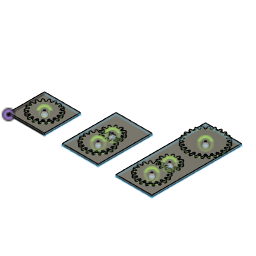
10-dimension-adjust-practice (Autodesk Fusion 360 design; units mm, degrees)
description: Spur Gear; Module: 2.000000; Num Teeth: 18; Pressure Angle: 20.000000; Backlash: 0.00 mm
description: Spur Gear; Module: 2.000000; Num Teeth: 12; Pressure Angle: 20.000000; Backlash: 0.00 mm
description: Spur Gear; Module: 2.000000; Num Teeth: 24; Pressure Angle: 20.000000; Backlash: 0.00 mm
Autodesk Fusion 360 part; units mm, degrees
sketch "スケッチ1" plane through (0, 0, 0) normal (0, 1, 0) x (1, 0, 0)
  line L0 (0, 0) -> (50, 0)
  line L1 (50, 0) -> (50, 50)
  line L2 (50, 50) -> (0, 50)
  line L3 (0, 50) -> (0, 0)
  circle A0 centre (25, 25) radius 1
  line L4 (75, 0) -> (125, 0)
  line L5 (125, 0) -> (125, 75)
  line L6 (125, 75) -> (75, 75)
  line L7 (75, 75) -> (75, 0)
  line L8 (150, 0) -> (200, 0)
  line L9 (200, 0) -> (200, 125)
  line L10 (200, 125) -> (150, 125)
  line L11 (150, 125) -> (150, 0)
  circle A1 centre (100, 25) radius 1
  circle A2 centre (100, 45) radius 1
  circle A3 centre (175, 25) radius 1
  circle A4 centre (175, 50) radius 1
  circle A5 centre (175, 100) radius 1
  dimension "d1" = 2
  dimension "d4" = 2
  dimension "d5" = 2
  dimension "d6" = 2
  dimension "d7" = 2
  dimension "d8" = 2
  constraint horizontal L0
  constraint vertical L1
  constraint horizontal L2
  constraint vertical L3
  constraint coincident L0.start L3.end
  constraint horizontal L4
  constraint vertical L5
  constraint horizontal L6
  constraint vertical L7
  constraint horizontal L8
  constraint vertical L9
  constraint horizontal L10
  constraint vertical L11
  measures "d1" diameter of A0
  measures "d4" diameter of A1
  measures "d5" diameter of A2
  measures "d6" diameter of A3
  measures "d7" diameter of A4
  measures "d8" diameter of A5
extrude "押し出し1" add sketch "スケッチ1" along normal blind 2.5 makes body 1 at (24.9751, 0, -41.9991) makes body 2 at (99.985, 0, -65.333) makes body 3 at (158.0114, 0, -58.4196)
cylinder "円柱プリミティブ2" add diameter 2 height 5 placed x (1, 0, 0) y (0, 0, -1) z (0, 1, 0) at (0, 0, -55) separate body makes body 4
copy_body "ボディ -> コンポーネント1" bodies 1 removing the originals makes body 5 in component "土台1"
copy_body "ボディ -> コンポーネント3" bodies 4 removing the originals makes body 6 in component "軸1"
sketch "スケッチ1 (2)" plane through (0, 0, 0) normal (0, 0, 1) x (1, 0, 0) in component "Spur Gear (18 teeth)"
  circle A0 centre (0, 0) radius 15.5492
  circle A1 centre (0, 0) radius 1
extrude "押し出し1'" add sketch "スケッチ1 (2)" along normal blind 2.5 separate body makes body 7 in component "Spur Gear (18 teeth)"
sketch "スケッチ2" plane through (0, 0, 0) normal (0, 0, 1) x (1, 0, 0) in component "Spur Gear (18 teeth)"
  spline S0 degree 5 poles (16.8263, -1.7252) (16.8353, -1.7261) (16.8534, -1.7277) (16.8805, -1.7293) (16.9168, -1.7301) (16.9623, -1.7292) (17.0078, -1.7268) (17.0533, -1.7236) (17.0989, -1.7199) (17.1446, -1.7159) (17.1902, -1.7115) (17.2359, -1.7067) (17.2816, -1.7013) (17.3273, -1.6953) (17.373, -1.6885) (17.4187, -1.6812) (17.4644, -1.6733) (17.5101, -1.6649) (17.5558, -1.6561) (17.6016, -1.647) (17.6473, -1.6374) (17.693, -1.6275) (17.7387, -1.6172) (17.7844, -1.6064) (17.8301, -1.5952) (17.8757, -1.5836) (17.9214, -1.5716) (17.967, -1.5592) (18.0127, -1.5465) (18.0583, -1.5335) (18.1039, -1.5201) (18.1494, -1.5063) (18.195, -1.4922) (18.2405, -1.4777) (18.286, -1.463) (18.3315, -1.4478) (18.377, -1.4324) (18.4224, -1.4166) (18.4678, -1.4005) (18.5132, -1.3841) (18.5585, -1.3674) (18.6038, -1.3503) (18.6491, -1.333) (18.6943, -1.3153) (18.7396, -1.2974) (18.7847, -1.2791) (18.8299, -1.2606) (18.875, -1.2418) (18.9201, -1.2226) (18.9651, -1.2032) (19.0101, -1.1835) (19.055, -1.1635) (19.1, -1.1433) (19.1448, -1.1227) (19.1897, -1.1019) (19.2344, -1.0808) (19.2792, -1.0594) (19.3239, -1.0378) (19.3685, -1.0159) (19.4131, -0.9937) (19.4577, -0.9712) (19.5022, -0.9485) (19.5467, -0.9255) (19.5911, -0.9023) (19.6354, -0.8788) (19.6797, -0.855) (19.724, -0.831) (19.7682, -0.8067) (19.8123, -0.7822) (19.8564, -0.7574) (19.9005, -0.7324) (19.9357, -0.7122) (19.962, -0.6969) (19.9796, -0.6867) (19.9884, -0.6815) knots 0 0 0 0 0 0 0.01428571 0.02857143 0.04285714 0.05714286 0.07142857 0.08571429 0.1 0.11428571 0.12857143 0.14285714 0.15714286 0.17142857 0.18571429 0.2 0.21428571 0.22857143 0.24285714 0.25714286 0.27142857 0.28571429 0.3 0.31428571 0.32857143 0.34285714 0.35714286 0.37142857 0.38571429 0.4 0.41428571 0.42857143 0.44285714 0.45714286 0.47142857 0.48571429 0.5 0.51428571 0.52857143 0.54285714 0.55714286 0.57142857 0.58571429 0.6 0.61428571 0.62857143 0.64285714 0.65714286 0.67142857 0.68571429 0.7 0.71428571 0.72857143 0.74285714 0.75714286 0.77142857 0.78571429 0.8 0.81428571 0.82857143 0.84285714 0.85714286 0.87142857 0.88571429 0.9 0.91428571 0.92857143 0.94285714 0.95714286 0.97142857 0.98571429 1 1 1 1 1 1
  spline S1 degree 5 poles (16.8263, 1.7252) (16.8353, 1.7261) (16.8534, 1.7277) (16.8805, 1.7293) (16.9168, 1.7301) (16.9623, 1.7292) (17.0078, 1.7268) (17.0533, 1.7236) (17.0989, 1.7199) (17.1446, 1.7159) (17.1902, 1.7115) (17.2359, 1.7067) (17.2816, 1.7013) (17.3273, 1.6953) (17.373, 1.6885) (17.4187, 1.6812) (17.4644, 1.6733) (17.5101, 1.6649) (17.5558, 1.6561) (17.6016, 1.647) (17.6473, 1.6374) (17.693, 1.6275) (17.7387, 1.6172) (17.7844, 1.6064) (17.8301, 1.5952) (17.8757, 1.5836) (17.9214, 1.5716) (17.967, 1.5592) (18.0127, 1.5465) (18.0583, 1.5335) (18.1039, 1.5201) (18.1494, 1.5063) (18.195, 1.4922) (18.2405, 1.4777) (18.286, 1.463) (18.3315, 1.4478) (18.377, 1.4324) (18.4224, 1.4166) (18.4678, 1.4005) (18.5132, 1.3841) (18.5585, 1.3674) (18.6038, 1.3503) (18.6491, 1.333) (18.6943, 1.3153) (18.7396, 1.2974) (18.7847, 1.2791) (18.8299, 1.2606) (18.875, 1.2418) (18.9201, 1.2226) (18.9651, 1.2032) (19.0101, 1.1835) (19.055, 1.1635) (19.1, 1.1433) (19.1448, 1.1227) (19.1897, 1.1019) (19.2344, 1.0808) (19.2792, 1.0594) (19.3239, 1.0378) (19.3685, 1.0159) (19.4131, 0.9937) (19.4577, 0.9712) (19.5022, 0.9485) (19.5467, 0.9255) (19.5911, 0.9023) (19.6354, 0.8788) (19.6797, 0.855) (19.724, 0.831) (19.7682, 0.8067) (19.8123, 0.7822) (19.8564, 0.7574) (19.9005, 0.7324) (19.9357, 0.7122) (19.962, 0.6969) (19.9796, 0.6867) (19.9884, 0.6815) knots 0 0 0 0 0 0 0.01428571 0.02857143 0.04285714 0.05714286 0.07142857 0.08571429 0.1 0.11428571 0.12857143 0.14285714 0.15714286 0.17142857 0.18571429 0.2 0.21428571 0.22857143 0.24285714 0.25714286 0.27142857 0.28571429 0.3 0.31428571 0.32857143 0.34285714 0.35714286 0.37142857 0.38571429 0.4 0.41428571 0.42857143 0.44285714 0.45714286 0.47142857 0.48571429 0.5 0.51428571 0.52857143 0.54285714 0.55714286 0.57142857 0.58571429 0.6 0.61428571 0.62857143 0.64285714 0.65714286 0.67142857 0.68571429 0.7 0.71428571 0.72857143 0.74285714 0.75714286 0.77142857 0.78571429 0.8 0.81428571 0.82857143 0.84285714 0.85714286 0.87142857 0.88571429 0.9 0.91428571 0.92857143 0.94285714 0.95714286 0.97142857 0.98571429 1 1 1 1 1 1
  arc A0 (19.9884, -0.6815) -> (19.9884, 0.6815) centre (0, 0) ccw
  line L0 (15.4582, -1.5859) -> (16.8263, -1.7252)
  line L1 (15.4582, 1.5859) -> (16.8263, 1.7252)
  line L2 (15.4582, -1.5859) -> (15.4582, 1.5859)
  point P0 (17.0479, -1.7239)
  point P1 (17.2716, -1.7024)
  point P2 (17.4964, -1.6673)
  point P3 (17.7221, -1.6209)
  point P4 (17.9484, -1.5642)
  point P5 (18.1752, -1.4983)
  point P6 (18.4023, -1.4236)
  point P7 (18.6295, -1.3405)
  point P8 (18.8567, -1.2494)
  point P9 (19.0838, -1.1505)
  point P10 (19.3106, -1.0442)
  point P11 (19.5371, -0.9304)
  point P12 (19.763, -0.8095)
  point P13 (17.0479, 1.7239)
  point P14 (17.2716, 1.7024)
  point P15 (17.4964, 1.6673)
  point P16 (17.7221, 1.6209)
  point P17 (17.9484, 1.5642)
  point P18 (18.1752, 1.4983)
  point P19 (18.4023, 1.4236)
  point P20 (18.6295, 1.3405)
  point P21 (18.8567, 1.2494)
  point P22 (19.0838, 1.1505)
  point P23 (19.3106, 1.0442)
  point P24 (19.5371, 0.9304)
  point P25 (19.763, 0.8095)
extrude "押し出し2" add sketch "スケッチ2" along normal blind 2.5 bodies 7 in component "Spur Gear (18 teeth)"
fillet "フィレット1" radius 1 2 edges at (15.468, -1.5869, 1.25) (15.468, 1.5869, 1.25) on bodies 7 in component "Spur Gear (18 teeth)"
pattern_circular "C パターン1" count 18 over 360 about axis through (0, 0, 0) along (0, 0, 1) of "押し出し2", "フィレット1" in component "Spur Gear (18 teeth)"
sketch "スケッチ3" plane through (0, 0, 0) normal (0, 0, 1) x (1, 0, 0) in component "Spur Gear (18 teeth)"
  circle A0 centre (0, 0) radius 18 construction
cylinder "円柱プリミティブ3" add diameter 2 height 5 placed x (1, 0, 0) y (0, 0, -1) z (0, 1, 0) at (75, 0, -80) separate body makes body 8
copy_body "ボディ -> コンポーネント4" bodies 2 removing the originals makes body 9 in component "土台2"
copy_body "ボディ -> コンポーネント5" bodies 8 removing the originals makes body 10 in component "軸2"
sketch "スケッチ1 (3)" plane through (0, 0, 0) normal (0, 0, 1) x (1, 0, 0) in component "Spur Gear (18 teeth) (1)"
  circle A0 centre (0, 0) radius 15.5492
  circle A1 centre (0, 0) radius 1
extrude "押し出し1''" add sketch "スケッチ1 (3)" along normal blind 2.5 separate body makes body 11 in component "Spur Gear (18 teeth) (1)"
sketch "スケッチ2 (2)" plane through (0, 0, 0) normal (0, 0, 1) x (1, 0, 0) in component "Spur Gear (18 teeth) (1)"
  spline S0 degree 5 poles (16.8263, -1.7252) (16.8353, -1.7261) (16.8534, -1.7277) (16.8805, -1.7293) (16.9168, -1.7301) (16.9623, -1.7292) (17.0078, -1.7268) (17.0533, -1.7236) (17.0989, -1.7199) (17.1446, -1.7159) (17.1902, -1.7115) (17.2359, -1.7067) (17.2816, -1.7013) (17.3273, -1.6953) (17.373, -1.6885) (17.4187, -1.6812) (17.4644, -1.6733) (17.5101, -1.6649) (17.5558, -1.6561) (17.6016, -1.647) (17.6473, -1.6374) (17.693, -1.6275) (17.7387, -1.6172) (17.7844, -1.6064) (17.8301, -1.5952) (17.8757, -1.5836) (17.9214, -1.5716) (17.967, -1.5592) (18.0127, -1.5465) (18.0583, -1.5335) (18.1039, -1.5201) (18.1494, -1.5063) (18.195, -1.4922) (18.2405, -1.4777) (18.286, -1.463) (18.3315, -1.4478) (18.377, -1.4324) (18.4224, -1.4166) (18.4678, -1.4005) (18.5132, -1.3841) (18.5585, -1.3674) (18.6038, -1.3503) (18.6491, -1.333) (18.6943, -1.3153) (18.7396, -1.2974) (18.7847, -1.2791) (18.8299, -1.2606) (18.875, -1.2418) (18.9201, -1.2226) (18.9651, -1.2032) (19.0101, -1.1835) (19.055, -1.1635) (19.1, -1.1433) (19.1448, -1.1227) (19.1897, -1.1019) (19.2344, -1.0808) (19.2792, -1.0594) (19.3239, -1.0378) (19.3685, -1.0159) (19.4131, -0.9937) (19.4577, -0.9712) (19.5022, -0.9485) (19.5467, -0.9255) (19.5911, -0.9023) (19.6354, -0.8788) (19.6797, -0.855) (19.724, -0.831) (19.7682, -0.8067) (19.8123, -0.7822) (19.8564, -0.7574) (19.9005, -0.7324) (19.9357, -0.7122) (19.962, -0.6969) (19.9796, -0.6867) (19.9884, -0.6815) knots 0 0 0 0 0 0 0.01428571 0.02857143 0.04285714 0.05714286 0.07142857 0.08571429 0.1 0.11428571 0.12857143 0.14285714 0.15714286 0.17142857 0.18571429 0.2 0.21428571 0.22857143 0.24285714 0.25714286 0.27142857 0.28571429 0.3 0.31428571 0.32857143 0.34285714 0.35714286 0.37142857 0.38571429 0.4 0.41428571 0.42857143 0.44285714 0.45714286 0.47142857 0.48571429 0.5 0.51428571 0.52857143 0.54285714 0.55714286 0.57142857 0.58571429 0.6 0.61428571 0.62857143 0.64285714 0.65714286 0.67142857 0.68571429 0.7 0.71428571 0.72857143 0.74285714 0.75714286 0.77142857 0.78571429 0.8 0.81428571 0.82857143 0.84285714 0.85714286 0.87142857 0.88571429 0.9 0.91428571 0.92857143 0.94285714 0.95714286 0.97142857 0.98571429 1 1 1 1 1 1
  spline S1 degree 5 poles (16.8263, 1.7252) (16.8353, 1.7261) (16.8534, 1.7277) (16.8805, 1.7293) (16.9168, 1.7301) (16.9623, 1.7292) (17.0078, 1.7268) (17.0533, 1.7236) (17.0989, 1.7199) (17.1446, 1.7159) (17.1902, 1.7115) (17.2359, 1.7067) (17.2816, 1.7013) (17.3273, 1.6953) (17.373, 1.6885) (17.4187, 1.6812) (17.4644, 1.6733) (17.5101, 1.6649) (17.5558, 1.6561) (17.6016, 1.647) (17.6473, 1.6374) (17.693, 1.6275) (17.7387, 1.6172) (17.7844, 1.6064) (17.8301, 1.5952) (17.8757, 1.5836) (17.9214, 1.5716) (17.967, 1.5592) (18.0127, 1.5465) (18.0583, 1.5335) (18.1039, 1.5201) (18.1494, 1.5063) (18.195, 1.4922) (18.2405, 1.4777) (18.286, 1.463) (18.3315, 1.4478) (18.377, 1.4324) (18.4224, 1.4166) (18.4678, 1.4005) (18.5132, 1.3841) (18.5585, 1.3674) (18.6038, 1.3503) (18.6491, 1.333) (18.6943, 1.3153) (18.7396, 1.2974) (18.7847, 1.2791) (18.8299, 1.2606) (18.875, 1.2418) (18.9201, 1.2226) (18.9651, 1.2032) (19.0101, 1.1835) (19.055, 1.1635) (19.1, 1.1433) (19.1448, 1.1227) (19.1897, 1.1019) (19.2344, 1.0808) (19.2792, 1.0594) (19.3239, 1.0378) (19.3685, 1.0159) (19.4131, 0.9937) (19.4577, 0.9712) (19.5022, 0.9485) (19.5467, 0.9255) (19.5911, 0.9023) (19.6354, 0.8788) (19.6797, 0.855) (19.724, 0.831) (19.7682, 0.8067) (19.8123, 0.7822) (19.8564, 0.7574) (19.9005, 0.7324) (19.9357, 0.7122) (19.962, 0.6969) (19.9796, 0.6867) (19.9884, 0.6815) knots 0 0 0 0 0 0 0.01428571 0.02857143 0.04285714 0.05714286 0.07142857 0.08571429 0.1 0.11428571 0.12857143 0.14285714 0.15714286 0.17142857 0.18571429 0.2 0.21428571 0.22857143 0.24285714 0.25714286 0.27142857 0.28571429 0.3 0.31428571 0.32857143 0.34285714 0.35714286 0.37142857 0.38571429 0.4 0.41428571 0.42857143 0.44285714 0.45714286 0.47142857 0.48571429 0.5 0.51428571 0.52857143 0.54285714 0.55714286 0.57142857 0.58571429 0.6 0.61428571 0.62857143 0.64285714 0.65714286 0.67142857 0.68571429 0.7 0.71428571 0.72857143 0.74285714 0.75714286 0.77142857 0.78571429 0.8 0.81428571 0.82857143 0.84285714 0.85714286 0.87142857 0.88571429 0.9 0.91428571 0.92857143 0.94285714 0.95714286 0.97142857 0.98571429 1 1 1 1 1 1
  arc A0 (19.9884, -0.6815) -> (19.9884, 0.6815) centre (0, 0) ccw
  line L0 (15.4582, -1.5859) -> (16.8263, -1.7252)
  line L1 (15.4582, 1.5859) -> (16.8263, 1.7252)
  line L2 (15.4582, -1.5859) -> (15.4582, 1.5859)
  point P0 (17.0479, -1.7239)
  point P1 (17.2716, -1.7024)
  point P2 (17.4964, -1.6673)
  point P3 (17.7221, -1.6209)
  point P4 (17.9484, -1.5642)
  point P5 (18.1752, -1.4983)
  point P6 (18.4023, -1.4236)
  point P7 (18.6295, -1.3405)
  point P8 (18.8567, -1.2494)
  point P9 (19.0838, -1.1505)
  point P10 (19.3106, -1.0442)
  point P11 (19.5371, -0.9304)
  point P12 (19.763, -0.8095)
  point P13 (17.0479, 1.7239)
  point P14 (17.2716, 1.7024)
  point P15 (17.4964, 1.6673)
  point P16 (17.7221, 1.6209)
  point P17 (17.9484, 1.5642)
  point P18 (18.1752, 1.4983)
  point P19 (18.4023, 1.4236)
  point P20 (18.6295, 1.3405)
  point P21 (18.8567, 1.2494)
  point P22 (19.0838, 1.1505)
  point P23 (19.3106, 1.0442)
  point P24 (19.5371, 0.9304)
  point P25 (19.763, 0.8095)
extrude "押し出し2'" add sketch "スケッチ2 (2)" along normal blind 2.5 bodies 11 in component "Spur Gear (18 teeth) (1)"
fillet "フィレット1'" radius 1 2 edges at (15.468, -1.5869, 1.25) (15.468, 1.5869, 1.25) on bodies 11 in component "Spur Gear (18 teeth) (1)"
pattern_circular "C パターン1'" count 18 over 360 about axis through (0, 0, 0) along (0, 0, 1) of "押し出し2'", "フィレット1'" in component "Spur Gear (18 teeth) (1)"
sketch "スケッチ3 (2)" plane through (0, 0, 0) normal (0, 0, 1) x (1, 0, 0) in component "Spur Gear (18 teeth) (1)"
  circle A0 centre (0, 0) radius 18 construction
sketch "スケッチ1 (4)" plane through (0, 0, 0) normal (0, 0, 1) x (1, 0, 0) in component "Spur Gear (12 teeth)"
  circle A0 centre (0, 0) radius 9.5492
  circle A1 centre (0, 0) radius 1
extrude "押し出し1'''" add sketch "スケッチ1 (4)" along normal blind 2.5 separate body makes body 12 in component "Spur Gear (12 teeth)"
sketch "スケッチ2 (3)" plane through (0, 0, 0) normal (0, 0, 1) x (1, 0, 0) in component "Spur Gear (12 teeth)"
  spline S0 degree 5 poles (11.1567, -1.6383) (11.1647, -1.6395) (11.1807, -1.6416) (11.2048, -1.6439) (11.237, -1.6456) (11.2774, -1.6458) (11.318, -1.6445) (11.3587, -1.6423) (11.3994, -1.6396) (11.4401, -1.6366) (11.4809, -1.6333) (11.5218, -1.6295) (11.5626, -1.625) (11.6035, -1.6199) (11.6445, -1.614) (11.6854, -1.6075) (11.7264, -1.6005) (11.7674, -1.5929) (11.8084, -1.585) (11.8494, -1.5766) (11.8905, -1.5678) (11.9315, -1.5587) (11.9725, -1.5491) (12.0135, -1.539) (12.0545, -1.5285) (12.0956, -1.5175) (12.1366, -1.5062) (12.1776, -1.4944) (12.2186, -1.4823) (12.2595, -1.4698) (12.3005, -1.4569) (12.3414, -1.4437) (12.3824, -1.4301) (12.4233, -1.4161) (12.4641, -1.4018) (12.505, -1.3871) (12.5458, -1.372) (12.5866, -1.3566) (12.6274, -1.3409) (12.6681, -1.3248) (12.7088, -1.3084) (12.7495, -1.2917) (12.7902, -1.2746) (12.8308, -1.2572) (12.8713, -1.2395) (12.9119, -1.2215) (12.9523, -1.2031) (12.9928, -1.1844) (13.0332, -1.1654) (13.0735, -1.1461) (13.1138, -1.1265) (13.1541, -1.1066) (13.1943, -1.0863) (13.2345, -1.0658) (13.2746, -1.045) (13.3146, -1.0239) (13.3546, -1.0024) (13.3946, -0.9807) (13.4344, -0.9587) (13.4743, -0.9364) (13.514, -0.9138) (13.5538, -0.8909) (13.5934, -0.8678) (13.633, -0.8443) (13.6725, -0.8206) (13.712, -0.7966) (13.7514, -0.7723) (13.7907, -0.7477) (13.8299, -0.7229) (13.8691, -0.6978) (13.9082, -0.6724) (13.9395, -0.6518) (13.9629, -0.6363) (13.9784, -0.6259) (13.9862, -0.6207) knots 0 0 0 0 0 0 0.01428571 0.02857143 0.04285714 0.05714286 0.07142857 0.08571429 0.1 0.11428571 0.12857143 0.14285714 0.15714286 0.17142857 0.18571429 0.2 0.21428571 0.22857143 0.24285714 0.25714286 0.27142857 0.28571429 0.3 0.31428571 0.32857143 0.34285714 0.35714286 0.37142857 0.38571429 0.4 0.41428571 0.42857143 0.44285714 0.45714286 0.47142857 0.48571429 0.5 0.51428571 0.52857143 0.54285714 0.55714286 0.57142857 0.58571429 0.6 0.61428571 0.62857143 0.64285714 0.65714286 0.67142857 0.68571429 0.7 0.71428571 0.72857143 0.74285714 0.75714286 0.77142857 0.78571429 0.8 0.81428571 0.82857143 0.84285714 0.85714286 0.87142857 0.88571429 0.9 0.91428571 0.92857143 0.94285714 0.95714286 0.97142857 0.98571429 1 1 1 1 1 1
  spline S1 degree 5 poles (11.1567, 1.6383) (11.1647, 1.6395) (11.1807, 1.6416) (11.2048, 1.6439) (11.237, 1.6456) (11.2774, 1.6458) (11.318, 1.6445) (11.3587, 1.6423) (11.3994, 1.6396) (11.4401, 1.6366) (11.4809, 1.6333) (11.5218, 1.6295) (11.5626, 1.625) (11.6035, 1.6199) (11.6445, 1.614) (11.6854, 1.6075) (11.7264, 1.6005) (11.7674, 1.5929) (11.8084, 1.585) (11.8494, 1.5766) (11.8905, 1.5678) (11.9315, 1.5587) (11.9725, 1.5491) (12.0135, 1.539) (12.0545, 1.5285) (12.0956, 1.5175) (12.1366, 1.5062) (12.1776, 1.4944) (12.2186, 1.4823) (12.2595, 1.4698) (12.3005, 1.4569) (12.3414, 1.4437) (12.3824, 1.4301) (12.4233, 1.4161) (12.4641, 1.4018) (12.505, 1.3871) (12.5458, 1.372) (12.5866, 1.3566) (12.6274, 1.3409) (12.6681, 1.3248) (12.7088, 1.3084) (12.7495, 1.2917) (12.7902, 1.2746) (12.8308, 1.2572) (12.8713, 1.2395) (12.9119, 1.2215) (12.9523, 1.2031) (12.9928, 1.1844) (13.0332, 1.1654) (13.0735, 1.1461) (13.1138, 1.1265) (13.1541, 1.1066) (13.1943, 1.0863) (13.2345, 1.0658) (13.2746, 1.045) (13.3146, 1.0239) (13.3546, 1.0024) (13.3946, 0.9807) (13.4344, 0.9587) (13.4743, 0.9364) (13.514, 0.9138) (13.5538, 0.8909) (13.5934, 0.8678) (13.633, 0.8443) (13.6725, 0.8206) (13.712, 0.7966) (13.7514, 0.7723) (13.7907, 0.7477) (13.8299, 0.7229) (13.8691, 0.6978) (13.9082, 0.6724) (13.9395, 0.6518) (13.9629, 0.6363) (13.9784, 0.6259) (13.9862, 0.6207) knots 0 0 0 0 0 0 0.01428571 0.02857143 0.04285714 0.05714286 0.07142857 0.08571429 0.1 0.11428571 0.12857143 0.14285714 0.15714286 0.17142857 0.18571429 0.2 0.21428571 0.22857143 0.24285714 0.25714286 0.27142857 0.28571429 0.3 0.31428571 0.32857143 0.34285714 0.35714286 0.37142857 0.38571429 0.4 0.41428571 0.42857143 0.44285714 0.45714286 0.47142857 0.48571429 0.5 0.51428571 0.52857143 0.54285714 0.55714286 0.57142857 0.58571429 0.6 0.61428571 0.62857143 0.64285714 0.65714286 0.67142857 0.68571429 0.7 0.71428571 0.72857143 0.74285714 0.75714286 0.77142857 0.78571429 0.8 0.81428571 0.82857143 0.84285714 0.85714286 0.87142857 0.88571429 0.9 0.91428571 0.92857143 0.94285714 0.95714286 0.97142857 0.98571429 1 1 1 1 1 1
  arc A0 (13.9862, -0.6207) -> (13.9862, 0.6207) centre (0, 0) ccw
  line L0 (9.438, -1.3874) -> (11.1567, -1.6383)
  line L1 (9.438, 1.3874) -> (11.1567, 1.6383)
  line L2 (9.438, -1.3874) -> (9.438, 1.3874)
  point P0 (11.3527, -1.6425)
  point P1 (11.5515, -1.6261)
  point P2 (11.7521, -1.5957)
  point P3 (11.954, -1.5533)
  point P4 (12.1568, -1.5003)
  point P5 (12.3603, -1.4374)
  point P6 (12.5642, -1.3651)
  point P7 (12.7683, -1.2838)
  point P8 (12.9724, -1.1938)
  point P9 (13.1764, -1.0953)
  point P10 (13.3799, -0.9887)
  point P11 (13.5828, -0.8739)
  point P12 (13.785, -0.7512)
  point P13 (11.3527, 1.6425)
  point P14 (11.5515, 1.6261)
  point P15 (11.7521, 1.5957)
  point P16 (11.954, 1.5533)
  point P17 (12.1568, 1.5003)
  point P18 (12.3603, 1.4374)
  point P19 (12.5642, 1.3651)
  point P20 (12.7683, 1.2838)
  point P21 (12.9724, 1.1938)
  point P22 (13.1764, 1.0953)
  point P23 (13.3799, 0.9887)
  point P24 (13.5828, 0.8739)
  point P25 (13.785, 0.7512)
extrude "押し出し2''" add sketch "スケッチ2 (3)" along normal blind 2.5 bodies 12 in component "Spur Gear (12 teeth)"
fillet "フィレット1''" radius 1 2 edges at (9.4477, -1.3888, 1.25) (9.4477, 1.3888, 1.25) on bodies 12 in component "Spur Gear (12 teeth)"
pattern_circular "C パターン1''" count 12 over 360 about axis through (0, 0, 0) along (0, 0, 1) of "押し出し2''", "フィレット1''" in component "Spur Gear (12 teeth)"
sketch "スケッチ3 (3)" plane through (0, 0, 0) normal (0, 0, 1) x (1, 0, 0) in component "Spur Gear (12 teeth)"
  circle A0 centre (0, 0) radius 12 construction
cylinder "円柱プリミティブ4" add diameter 2 height 5 placed x (1, 0, 0) y (0, 0, -1) z (0, 1, 0) at (150, 0, -130) separate body makes body 13
copy_body "ボディ -> コンポーネント7" bodies 13 removing the originals makes body 14 in component "軸3"
copy_body "ボディ -> コンポーネント8" bodies 3 removing the originals makes body 15 in component "土台3"
sketch "スケッチ1 (5)" plane through (0, 0, 0) normal (0, 0, 1) x (1, 0, 0) in component "Spur Gear (18 teeth) (2)"
  circle A0 centre (0, 0) radius 15.5492
  circle A1 centre (0, 0) radius 1
extrude "押し出し1''''" add sketch "スケッチ1 (5)" along normal blind 2.5 separate body makes body 16 in component "Spur Gear (18 teeth) (2)"
sketch "スケッチ2 (4)" plane through (0, 0, 0) normal (0, 0, 1) x (1, 0, 0) in component "Spur Gear (18 teeth) (2)"
  spline S0 degree 5 poles (16.8263, -1.7252) (16.8353, -1.7261) (16.8534, -1.7277) (16.8805, -1.7293) (16.9168, -1.7301) (16.9623, -1.7292) (17.0078, -1.7268) (17.0533, -1.7236) (17.0989, -1.7199) (17.1446, -1.7159) (17.1902, -1.7115) (17.2359, -1.7067) (17.2816, -1.7013) (17.3273, -1.6953) (17.373, -1.6885) (17.4187, -1.6812) (17.4644, -1.6733) (17.5101, -1.6649) (17.5558, -1.6561) (17.6016, -1.647) (17.6473, -1.6374) (17.693, -1.6275) (17.7387, -1.6172) (17.7844, -1.6064) (17.8301, -1.5952) (17.8757, -1.5836) (17.9214, -1.5716) (17.967, -1.5592) (18.0127, -1.5465) (18.0583, -1.5335) (18.1039, -1.5201) (18.1494, -1.5063) (18.195, -1.4922) (18.2405, -1.4777) (18.286, -1.463) (18.3315, -1.4478) (18.377, -1.4324) (18.4224, -1.4166) (18.4678, -1.4005) (18.5132, -1.3841) (18.5585, -1.3674) (18.6038, -1.3503) (18.6491, -1.333) (18.6943, -1.3153) (18.7396, -1.2974) (18.7847, -1.2791) (18.8299, -1.2606) (18.875, -1.2418) (18.9201, -1.2226) (18.9651, -1.2032) (19.0101, -1.1835) (19.055, -1.1635) (19.1, -1.1433) (19.1448, -1.1227) (19.1897, -1.1019) (19.2344, -1.0808) (19.2792, -1.0594) (19.3239, -1.0378) (19.3685, -1.0159) (19.4131, -0.9937) (19.4577, -0.9712) (19.5022, -0.9485) (19.5467, -0.9255) (19.5911, -0.9023) (19.6354, -0.8788) (19.6797, -0.855) (19.724, -0.831) (19.7682, -0.8067) (19.8123, -0.7822) (19.8564, -0.7574) (19.9005, -0.7324) (19.9357, -0.7122) (19.962, -0.6969) (19.9796, -0.6867) (19.9884, -0.6815) knots 0 0 0 0 0 0 0.01428571 0.02857143 0.04285714 0.05714286 0.07142857 0.08571429 0.1 0.11428571 0.12857143 0.14285714 0.15714286 0.17142857 0.18571429 0.2 0.21428571 0.22857143 0.24285714 0.25714286 0.27142857 0.28571429 0.3 0.31428571 0.32857143 0.34285714 0.35714286 0.37142857 0.38571429 0.4 0.41428571 0.42857143 0.44285714 0.45714286 0.47142857 0.48571429 0.5 0.51428571 0.52857143 0.54285714 0.55714286 0.57142857 0.58571429 0.6 0.61428571 0.62857143 0.64285714 0.65714286 0.67142857 0.68571429 0.7 0.71428571 0.72857143 0.74285714 0.75714286 0.77142857 0.78571429 0.8 0.81428571 0.82857143 0.84285714 0.85714286 0.87142857 0.88571429 0.9 0.91428571 0.92857143 0.94285714 0.95714286 0.97142857 0.98571429 1 1 1 1 1 1
  spline S1 degree 5 poles (16.8263, 1.7252) (16.8353, 1.7261) (16.8534, 1.7277) (16.8805, 1.7293) (16.9168, 1.7301) (16.9623, 1.7292) (17.0078, 1.7268) (17.0533, 1.7236) (17.0989, 1.7199) (17.1446, 1.7159) (17.1902, 1.7115) (17.2359, 1.7067) (17.2816, 1.7013) (17.3273, 1.6953) (17.373, 1.6885) (17.4187, 1.6812) (17.4644, 1.6733) (17.5101, 1.6649) (17.5558, 1.6561) (17.6016, 1.647) (17.6473, 1.6374) (17.693, 1.6275) (17.7387, 1.6172) (17.7844, 1.6064) (17.8301, 1.5952) (17.8757, 1.5836) (17.9214, 1.5716) (17.967, 1.5592) (18.0127, 1.5465) (18.0583, 1.5335) (18.1039, 1.5201) (18.1494, 1.5063) (18.195, 1.4922) (18.2405, 1.4777) (18.286, 1.463) (18.3315, 1.4478) (18.377, 1.4324) (18.4224, 1.4166) (18.4678, 1.4005) (18.5132, 1.3841) (18.5585, 1.3674) (18.6038, 1.3503) (18.6491, 1.333) (18.6943, 1.3153) (18.7396, 1.2974) (18.7847, 1.2791) (18.8299, 1.2606) (18.875, 1.2418) (18.9201, 1.2226) (18.9651, 1.2032) (19.0101, 1.1835) (19.055, 1.1635) (19.1, 1.1433) (19.1448, 1.1227) (19.1897, 1.1019) (19.2344, 1.0808) (19.2792, 1.0594) (19.3239, 1.0378) (19.3685, 1.0159) (19.4131, 0.9937) (19.4577, 0.9712) (19.5022, 0.9485) (19.5467, 0.9255) (19.5911, 0.9023) (19.6354, 0.8788) (19.6797, 0.855) (19.724, 0.831) (19.7682, 0.8067) (19.8123, 0.7822) (19.8564, 0.7574) (19.9005, 0.7324) (19.9357, 0.7122) (19.962, 0.6969) (19.9796, 0.6867) (19.9884, 0.6815) knots 0 0 0 0 0 0 0.01428571 0.02857143 0.04285714 0.05714286 0.07142857 0.08571429 0.1 0.11428571 0.12857143 0.14285714 0.15714286 0.17142857 0.18571429 0.2 0.21428571 0.22857143 0.24285714 0.25714286 0.27142857 0.28571429 0.3 0.31428571 0.32857143 0.34285714 0.35714286 0.37142857 0.38571429 0.4 0.41428571 0.42857143 0.44285714 0.45714286 0.47142857 0.48571429 0.5 0.51428571 0.52857143 0.54285714 0.55714286 0.57142857 0.58571429 0.6 0.61428571 0.62857143 0.64285714 0.65714286 0.67142857 0.68571429 0.7 0.71428571 0.72857143 0.74285714 0.75714286 0.77142857 0.78571429 0.8 0.81428571 0.82857143 0.84285714 0.85714286 0.87142857 0.88571429 0.9 0.91428571 0.92857143 0.94285714 0.95714286 0.97142857 0.98571429 1 1 1 1 1 1
  arc A0 (19.9884, -0.6815) -> (19.9884, 0.6815) centre (0, 0) ccw
  line L0 (15.4582, -1.5859) -> (16.8263, -1.7252)
  line L1 (15.4582, 1.5859) -> (16.8263, 1.7252)
  line L2 (15.4582, -1.5859) -> (15.4582, 1.5859)
  point P0 (17.0479, -1.7239)
  point P1 (17.2716, -1.7024)
  point P2 (17.4964, -1.6673)
  point P3 (17.7221, -1.6209)
  point P4 (17.9484, -1.5642)
  point P5 (18.1752, -1.4983)
  point P6 (18.4023, -1.4236)
  point P7 (18.6295, -1.3405)
  point P8 (18.8567, -1.2494)
  point P9 (19.0838, -1.1505)
  point P10 (19.3106, -1.0442)
  point P11 (19.5371, -0.9304)
  point P12 (19.763, -0.8095)
  point P13 (17.0479, 1.7239)
  point P14 (17.2716, 1.7024)
  point P15 (17.4964, 1.6673)
  point P16 (17.7221, 1.6209)
  point P17 (17.9484, 1.5642)
  point P18 (18.1752, 1.4983)
  point P19 (18.4023, 1.4236)
  point P20 (18.6295, 1.3405)
  point P21 (18.8567, 1.2494)
  point P22 (19.0838, 1.1505)
  point P23 (19.3106, 1.0442)
  point P24 (19.5371, 0.9304)
  point P25 (19.763, 0.8095)
extrude "押し出し2'''" add sketch "スケッチ2 (4)" along normal blind 2.5 bodies 16 in component "Spur Gear (18 teeth) (2)"
fillet "フィレット1'''" radius 1 2 edges at (15.468, -1.5869, 1.25) (15.468, 1.5869, 1.25) on bodies 16 in component "Spur Gear (18 teeth) (2)"
pattern_circular "C パターン1'''" count 18 over 360 about axis through (0, 0, 0) along (0, 0, 1) of "押し出し2'''", "フィレット1'''" in component "Spur Gear (18 teeth) (2)"
sketch "スケッチ3 (4)" plane through (0, 0, 0) normal (0, 0, 1) x (1, 0, 0) in component "Spur Gear (18 teeth) (2)"
  circle A0 centre (0, 0) radius 18 construction
sketch "スケッチ1 (6)" plane through (0, 0, 0) normal (0, 0, 1) x (1, 0, 0) in component "Spur Gear (12 teeth) (1)"
  circle A0 centre (0, 0) radius 9.5492
  circle A1 centre (0, 0) radius 1
extrude "押し出し1'''''" add sketch "スケッチ1 (6)" along normal blind 2.5 separate body makes body 17 in component "Spur Gear (12 teeth) (1)"
sketch "スケッチ2 (5)" plane through (0, 0, 0) normal (0, 0, 1) x (1, 0, 0) in component "Spur Gear (12 teeth) (1)"
  spline S0 degree 5 poles (11.1567, -1.6383) (11.1647, -1.6395) (11.1807, -1.6416) (11.2048, -1.6439) (11.237, -1.6456) (11.2774, -1.6458) (11.318, -1.6445) (11.3587, -1.6423) (11.3994, -1.6396) (11.4401, -1.6366) (11.4809, -1.6333) (11.5218, -1.6295) (11.5626, -1.625) (11.6035, -1.6199) (11.6445, -1.614) (11.6854, -1.6075) (11.7264, -1.6005) (11.7674, -1.5929) (11.8084, -1.585) (11.8494, -1.5766) (11.8905, -1.5678) (11.9315, -1.5587) (11.9725, -1.5491) (12.0135, -1.539) (12.0545, -1.5285) (12.0956, -1.5175) (12.1366, -1.5062) (12.1776, -1.4944) (12.2186, -1.4823) (12.2595, -1.4698) (12.3005, -1.4569) (12.3414, -1.4437) (12.3824, -1.4301) (12.4233, -1.4161) (12.4641, -1.4018) (12.505, -1.3871) (12.5458, -1.372) (12.5866, -1.3566) (12.6274, -1.3409) (12.6681, -1.3248) (12.7088, -1.3084) (12.7495, -1.2917) (12.7902, -1.2746) (12.8308, -1.2572) (12.8713, -1.2395) (12.9119, -1.2215) (12.9523, -1.2031) (12.9928, -1.1844) (13.0332, -1.1654) (13.0735, -1.1461) (13.1138, -1.1265) (13.1541, -1.1066) (13.1943, -1.0863) (13.2345, -1.0658) (13.2746, -1.045) (13.3146, -1.0239) (13.3546, -1.0024) (13.3946, -0.9807) (13.4344, -0.9587) (13.4743, -0.9364) (13.514, -0.9138) (13.5538, -0.8909) (13.5934, -0.8678) (13.633, -0.8443) (13.6725, -0.8206) (13.712, -0.7966) (13.7514, -0.7723) (13.7907, -0.7477) (13.8299, -0.7229) (13.8691, -0.6978) (13.9082, -0.6724) (13.9395, -0.6518) (13.9629, -0.6363) (13.9784, -0.6259) (13.9862, -0.6207) knots 0 0 0 0 0 0 0.01428571 0.02857143 0.04285714 0.05714286 0.07142857 0.08571429 0.1 0.11428571 0.12857143 0.14285714 0.15714286 0.17142857 0.18571429 0.2 0.21428571 0.22857143 0.24285714 0.25714286 0.27142857 0.28571429 0.3 0.31428571 0.32857143 0.34285714 0.35714286 0.37142857 0.38571429 0.4 0.41428571 0.42857143 0.44285714 0.45714286 0.47142857 0.48571429 0.5 0.51428571 0.52857143 0.54285714 0.55714286 0.57142857 0.58571429 0.6 0.61428571 0.62857143 0.64285714 0.65714286 0.67142857 0.68571429 0.7 0.71428571 0.72857143 0.74285714 0.75714286 0.77142857 0.78571429 0.8 0.81428571 0.82857143 0.84285714 0.85714286 0.87142857 0.88571429 0.9 0.91428571 0.92857143 0.94285714 0.95714286 0.97142857 0.98571429 1 1 1 1 1 1
  spline S1 degree 5 poles (11.1567, 1.6383) (11.1647, 1.6395) (11.1807, 1.6416) (11.2048, 1.6439) (11.237, 1.6456) (11.2774, 1.6458) (11.318, 1.6445) (11.3587, 1.6423) (11.3994, 1.6396) (11.4401, 1.6366) (11.4809, 1.6333) (11.5218, 1.6295) (11.5626, 1.625) (11.6035, 1.6199) (11.6445, 1.614) (11.6854, 1.6075) (11.7264, 1.6005) (11.7674, 1.5929) (11.8084, 1.585) (11.8494, 1.5766) (11.8905, 1.5678) (11.9315, 1.5587) (11.9725, 1.5491) (12.0135, 1.539) (12.0545, 1.5285) (12.0956, 1.5175) (12.1366, 1.5062) (12.1776, 1.4944) (12.2186, 1.4823) (12.2595, 1.4698) (12.3005, 1.4569) (12.3414, 1.4437) (12.3824, 1.4301) (12.4233, 1.4161) (12.4641, 1.4018) (12.505, 1.3871) (12.5458, 1.372) (12.5866, 1.3566) (12.6274, 1.3409) (12.6681, 1.3248) (12.7088, 1.3084) (12.7495, 1.2917) (12.7902, 1.2746) (12.8308, 1.2572) (12.8713, 1.2395) (12.9119, 1.2215) (12.9523, 1.2031) (12.9928, 1.1844) (13.0332, 1.1654) (13.0735, 1.1461) (13.1138, 1.1265) (13.1541, 1.1066) (13.1943, 1.0863) (13.2345, 1.0658) (13.2746, 1.045) (13.3146, 1.0239) (13.3546, 1.0024) (13.3946, 0.9807) (13.4344, 0.9587) (13.4743, 0.9364) (13.514, 0.9138) (13.5538, 0.8909) (13.5934, 0.8678) (13.633, 0.8443) (13.6725, 0.8206) (13.712, 0.7966) (13.7514, 0.7723) (13.7907, 0.7477) (13.8299, 0.7229) (13.8691, 0.6978) (13.9082, 0.6724) (13.9395, 0.6518) (13.9629, 0.6363) (13.9784, 0.6259) (13.9862, 0.6207) knots 0 0 0 0 0 0 0.01428571 0.02857143 0.04285714 0.05714286 0.07142857 0.08571429 0.1 0.11428571 0.12857143 0.14285714 0.15714286 0.17142857 0.18571429 0.2 0.21428571 0.22857143 0.24285714 0.25714286 0.27142857 0.28571429 0.3 0.31428571 0.32857143 0.34285714 0.35714286 0.37142857 0.38571429 0.4 0.41428571 0.42857143 0.44285714 0.45714286 0.47142857 0.48571429 0.5 0.51428571 0.52857143 0.54285714 0.55714286 0.57142857 0.58571429 0.6 0.61428571 0.62857143 0.64285714 0.65714286 0.67142857 0.68571429 0.7 0.71428571 0.72857143 0.74285714 0.75714286 0.77142857 0.78571429 0.8 0.81428571 0.82857143 0.84285714 0.85714286 0.87142857 0.88571429 0.9 0.91428571 0.92857143 0.94285714 0.95714286 0.97142857 0.98571429 1 1 1 1 1 1
  arc A0 (13.9862, -0.6207) -> (13.9862, 0.6207) centre (0, 0) ccw
  line L0 (9.438, -1.3874) -> (11.1567, -1.6383)
  line L1 (9.438, 1.3874) -> (11.1567, 1.6383)
  line L2 (9.438, -1.3874) -> (9.438, 1.3874)
  point P0 (11.3527, -1.6425)
  point P1 (11.5515, -1.6261)
  point P2 (11.7521, -1.5957)
  point P3 (11.954, -1.5533)
  point P4 (12.1568, -1.5003)
  point P5 (12.3603, -1.4374)
  point P6 (12.5642, -1.3651)
  point P7 (12.7683, -1.2838)
  point P8 (12.9724, -1.1938)
  point P9 (13.1764, -1.0953)
  point P10 (13.3799, -0.9887)
  point P11 (13.5828, -0.8739)
  point P12 (13.785, -0.7512)
  point P13 (11.3527, 1.6425)
  point P14 (11.5515, 1.6261)
  point P15 (11.7521, 1.5957)
  point P16 (11.954, 1.5533)
  point P17 (12.1568, 1.5003)
  point P18 (12.3603, 1.4374)
  point P19 (12.5642, 1.3651)
  point P20 (12.7683, 1.2838)
  point P21 (12.9724, 1.1938)
  point P22 (13.1764, 1.0953)
  point P23 (13.3799, 0.9887)
  point P24 (13.5828, 0.8739)
  point P25 (13.785, 0.7512)
extrude "押し出し2''''" add sketch "スケッチ2 (5)" along normal blind 2.5 bodies 17 in component "Spur Gear (12 teeth) (1)"
fillet "フィレット1''''" radius 1 2 edges at (9.4477, -1.3888, 1.25) (9.4477, 1.3888, 1.25) on bodies 17 in component "Spur Gear (12 teeth) (1)"
pattern_circular "C パターン1''''" count 12 over 360 about axis through (0, 0, 0) along (0, 0, 1) of "押し出し2''''", "フィレット1''''" in component "Spur Gear (12 teeth) (1)"
sketch "スケッチ3 (5)" plane through (0, 0, 0) normal (0, 0, 1) x (1, 0, 0) in component "Spur Gear (12 teeth) (1)"
  circle A0 centre (0, 0) radius 12 construction
sketch "スケッチ1 (7)" plane through (0, 0, 0) normal (0, 0, 1) x (1, 0, 0) in component "Spur Gear (24 teeth)"
  circle A0 centre (0, 0) radius 21.5492
  circle A1 centre (0, 0) radius 1
extrude "押し出し1''''''" add sketch "スケッチ1 (7)" along normal blind 2.5 separate body makes body 18 in component "Spur Gear (24 teeth)"
sketch "スケッチ2 (6)" plane through (0, 0, 0) normal (0, 0, 1) x (1, 0, 0) in component "Spur Gear (24 teeth)"
  spline S0 degree 5 poles (22.4799, -1.8102) (22.4899, -1.8111) (22.5101, -1.8124) (22.5404, -1.8137) (22.5808, -1.814) (22.6313, -1.8123) (22.6819, -1.8093) (22.7326, -1.8054) (22.7832, -1.801) (22.8339, -1.7962) (22.8846, -1.7911) (22.9353, -1.7856) (22.986, -1.7795) (23.0367, -1.7727) (23.0874, -1.7652) (23.1381, -1.7571) (23.1889, -1.7484) (23.2396, -1.7393) (23.2903, -1.7297) (23.341, -1.7198) (23.3916, -1.7095) (23.4423, -1.6988) (23.493, -1.6877) (23.5436, -1.6762) (23.5943, -1.6642) (23.6449, -1.6518) (23.6955, -1.6391) (23.7461, -1.6259) (23.7966, -1.6124) (23.8472, -1.5986) (23.8977, -1.5844) (23.9482, -1.5699) (23.9987, -1.555) (24.0491, -1.5398) (24.0996, -1.5242) (24.15, -1.5083) (24.2004, -1.4921) (24.2507, -1.4756) (24.301, -1.4587) (24.3513, -1.4415) (24.4016, -1.424) (24.4518, -1.4062) (24.502, -1.3881) (24.5522, -1.3697) (24.6024, -1.351) (24.6525, -1.3321) (24.7025, -1.3128) (24.7526, -1.2932) (24.8026, -1.2733) (24.8525, -1.2532) (24.9025, -1.2327) (24.9523, -1.212) (25.0022, -1.191) (25.052, -1.1697) (25.1018, -1.1482) (25.1515, -1.1264) (25.2012, -1.1043) (25.2509, -1.0819) (25.3005, -1.0593) (25.35, -1.0364) (25.3995, -1.0133) (25.449, -0.9898) (25.4985, -0.9662) (25.5478, -0.9422) (25.5972, -0.9181) (25.6465, -0.8936) (25.6957, -0.8689) (25.7449, -0.844) (25.7941, -0.8188) (25.8432, -0.7933) (25.8922, -0.7676) (25.9314, -0.7469) (25.9608, -0.7312) (25.9804, -0.7207) (25.9902, -0.7155) knots 0 0 0 0 0 0 0.01428571 0.02857143 0.04285714 0.05714286 0.07142857 0.08571429 0.1 0.11428571 0.12857143 0.14285714 0.15714286 0.17142857 0.18571429 0.2 0.21428571 0.22857143 0.24285714 0.25714286 0.27142857 0.28571429 0.3 0.31428571 0.32857143 0.34285714 0.35714286 0.37142857 0.38571429 0.4 0.41428571 0.42857143 0.44285714 0.45714286 0.47142857 0.48571429 0.5 0.51428571 0.52857143 0.54285714 0.55714286 0.57142857 0.58571429 0.6 0.61428571 0.62857143 0.64285714 0.65714286 0.67142857 0.68571429 0.7 0.71428571 0.72857143 0.74285714 0.75714286 0.77142857 0.78571429 0.8 0.81428571 0.82857143 0.84285714 0.85714286 0.87142857 0.88571429 0.9 0.91428571 0.92857143 0.94285714 0.95714286 0.97142857 0.98571429 1 1 1 1 1 1
  spline S1 degree 5 poles (22.4799, 1.8102) (22.4899, 1.8111) (22.5101, 1.8124) (22.5404, 1.8137) (22.5808, 1.814) (22.6313, 1.8123) (22.6819, 1.8093) (22.7326, 1.8054) (22.7832, 1.801) (22.8339, 1.7962) (22.8846, 1.7911) (22.9353, 1.7856) (22.986, 1.7795) (23.0367, 1.7727) (23.0874, 1.7652) (23.1381, 1.7571) (23.1889, 1.7484) (23.2396, 1.7393) (23.2903, 1.7297) (23.341, 1.7198) (23.3916, 1.7095) (23.4423, 1.6988) (23.493, 1.6877) (23.5436, 1.6762) (23.5943, 1.6642) (23.6449, 1.6518) (23.6955, 1.6391) (23.7461, 1.6259) (23.7966, 1.6124) (23.8472, 1.5986) (23.8977, 1.5844) (23.9482, 1.5699) (23.9987, 1.555) (24.0491, 1.5398) (24.0996, 1.5242) (24.15, 1.5083) (24.2004, 1.4921) (24.2507, 1.4756) (24.301, 1.4587) (24.3513, 1.4415) (24.4016, 1.424) (24.4518, 1.4062) (24.502, 1.3881) (24.5522, 1.3697) (24.6024, 1.351) (24.6525, 1.3321) (24.7025, 1.3128) (24.7526, 1.2932) (24.8026, 1.2733) (24.8525, 1.2532) (24.9025, 1.2327) (24.9523, 1.212) (25.0022, 1.191) (25.052, 1.1697) (25.1018, 1.1482) (25.1515, 1.1264) (25.2012, 1.1043) (25.2509, 1.0819) (25.3005, 1.0593) (25.35, 1.0364) (25.3995, 1.0133) (25.449, 0.9898) (25.4985, 0.9662) (25.5478, 0.9422) (25.5972, 0.9181) (25.6465, 0.8936) (25.6957, 0.8689) (25.7449, 0.844) (25.7941, 0.8188) (25.8432, 0.7933) (25.8922, 0.7676) (25.9314, 0.7469) (25.9608, 0.7312) (25.9804, 0.7207) (25.9902, 0.7155) knots 0 0 0 0 0 0 0.01428571 0.02857143 0.04285714 0.05714286 0.07142857 0.08571429 0.1 0.11428571 0.12857143 0.14285714 0.15714286 0.17142857 0.18571429 0.2 0.21428571 0.22857143 0.24285714 0.25714286 0.27142857 0.28571429 0.3 0.31428571 0.32857143 0.34285714 0.35714286 0.37142857 0.38571429 0.4 0.41428571 0.42857143 0.44285714 0.45714286 0.47142857 0.48571429 0.5 0.51428571 0.52857143 0.54285714 0.55714286 0.57142857 0.58571429 0.6 0.61428571 0.62857143 0.64285714 0.65714286 0.67142857 0.68571429 0.7 0.71428571 0.72857143 0.74285714 0.75714286 0.77142857 0.78571429 0.8 0.81428571 0.82857143 0.84285714 0.85714286 0.87142857 0.88571429 0.9 0.91428571 0.92857143 0.94285714 0.95714286 0.97142857 0.98571429 1 1 1 1 1 1
  arc A0 (25.9902, -0.7155) -> (25.9902, 0.7155) centre (0, 0) ccw
  line L0 (21.4697, -1.7297) -> (22.4799, -1.8102)
  line L1 (21.4697, 1.7297) -> (22.4799, 1.8102)
  line L2 (21.4697, -1.7297) -> (21.4697, 1.7297)
  point P0 (22.7272, -1.8057)
  point P1 (22.9762, -1.7806)
  point P2 (23.2261, -1.7416)
  point P3 (23.4768, -1.6912)
  point P4 (23.7279, -1.6306)
  point P5 (23.9793, -1.5607)
  point P6 (24.231, -1.482)
  point P7 (24.4828, -1.395)
  point P8 (24.7346, -1.3002)
  point P9 (24.9863, -1.1976)
  point P10 (25.2378, -1.0877)
  point P11 (25.489, -0.9706)
  point P12 (25.7398, -0.8465)
  point P13 (22.7272, 1.8057)
  point P14 (22.9762, 1.7806)
  point P15 (23.2261, 1.7416)
  point P16 (23.4768, 1.6912)
  point P17 (23.7279, 1.6306)
  point P18 (23.9793, 1.5607)
  point P19 (24.231, 1.482)
  point P20 (24.4828, 1.395)
  point P21 (24.7346, 1.3002)
  point P22 (24.9863, 1.1976)
  point P23 (25.2378, 1.0877)
  point P24 (25.489, 0.9706)
  point P25 (25.7398, 0.8465)
extrude "押し出し2'''''" add sketch "スケッチ2 (6)" along normal blind 2.5 bodies 18 in component "Spur Gear (24 teeth)"
fillet "フィレット1'''''" radius 1 2 edges at (21.4796, -1.7305, 1.25) (21.4796, 1.7305, 1.25) on bodies 18 in component "Spur Gear (24 teeth)"
pattern_circular "C パターン1'''''" count 24 over 360 about axis through (0, 0, 0) along (0, 0, 1) of "押し出し2'''''", "フィレット1'''''" in component "Spur Gear (24 teeth)"
sketch "スケッチ3 (6)" plane through (0, 0, 0) normal (0, 0, 1) x (1, 0, 0) in component "Spur Gear (24 teeth)"
  circle A0 centre (0, 0) radius 24 construction
component "ギア1" placed x (1, 0, 0) y (0, 1, 0) z (0, 0, 1) at (0, 0, 0)
component "ギア2" placed x (1, 0, 0) y (0, 1, 0) z (0, 0, 1) at (0, 0, 0)
component "ギア3" placed x (1, 0, 0) y (0, 1, 0) z (0, 0, 1) at (0, 0, 0)
component "軸3" placed x (1, 0, 0) y (0, 1, 0) z (0, 0, 1) at (25, 0, 105)
component "Spur Gear (18 teeth)" placed x (1, 0, 0) y (0, 0, -1) z (0, 1, 0) at (25, 2.5, -25) in component "ギア1"
component "軸1" placed x (1, 0, 0) y (0, 1, 0) z (0, 0, 1) at (25, 0, 30) in component "ギア1"
component "土台1" placed x (1, 0, 0) y (0, 1, 0) z (0, 0, 1) at (0, 0, 0) in component "ギア1"
component "土台2" placed x (1, 0, 0) y (0, 1, 0) z (0, 0, 1) at (0, 0, 0) in component "ギア2"
component "軸2" placed x (1, 0, 0) y (0, 1, 0) z (0, 0, 1) at (25, 0, 55) in component "ギア2"
component "軸2" placed x (1, 0, 0) y (0, 1, 0) z (0, 0, 1) at (25, 0, 35) in component "ギア2"
component "Spur Gear (18 teeth) (1)" placed x (1, 0, 0) y (0, 0, -1) z (0, 1, 0) at (100, 2.5, -25) in component "ギア2"
component "Spur Gear (12 teeth)" placed x (1, 0, 0) y (0, 0, -1) z (0, 1, 0) at (100, 2.5, -45) in component "ギア2"
component "軸3" placed x (1, 0, 0) y (0, 1, 0) z (0, 0, 1) at (25, 0, 30) in component "ギア3"
component "土台3" placed x (1, 0, 0) y (0, 1, 0) z (0, 0, 1) at (0, 0, 0) in component "ギア3"
component "軸3" placed x (1, 0, 0) y (0, 1, 0) z (0, 0, 1) at (25, 0, 80) in component "ギア3"
component "Spur Gear (18 teeth) (2)" placed x (1, 0, 0) y (0, 0, -1) z (0, 1, 0) at (175, 2.5, -25) in component "ギア3"
component "Spur Gear (12 teeth) (1)" placed x (1, 0, 0) y (0, 0, -1) z (0, 1, 0) at (175, 2.5, -50) in component "ギア3"
component "Spur Gear (24 teeth)" placed x (0.991445, 0, -0.130526) y (-0.130526, 0, -0.991445) z (0, 1, 0) at (175, 2.5, -100) in component "ギア3"
named bodies: "土台3", "軸2"
